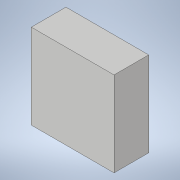
# Autodesk Inventor part: Battery
Saved by Autodesk Inventor 2021 (Build 250183000, 183)
## iProperties
Created: 2020-10-20
Part Number: Battery
Material: Generic
Document SubType Name: Modeling
Designer: Jawal
Density: 1 g/cm^3
Appearance: Default
Author: Jawal
Autodesk Inventor part; units mm, degrees
ref_plane "YZ Plane" through (0, 0, 0) normal (1, 0, 0) x (0, 1, 0)
ref_plane "XZ Plane" through (0, 0, 0) normal (0, 1, 0) x (-1, 0, 0)
ref_plane "XY Plane" through (0, 0, 0) normal (0, 0, 1) x (1, 0, 0)
sketch "Sketch2" plane through (0, 0, 0) normal (0, 0, 1) x (1, 0, 0)
  line L0 (0, 0) -> (135, 0)
  line L1 (135, 0) -> (135, 139)
  line L2 (135, 139) -> (0, 139)
  line L3 (0, 139) -> (0, 0)
  dimension "d4" = 135
  dimension "d5" = 139
  constraints: 8 end point, 2 parallel, 1 horizontal, 1 perpendicular
  measures "d4" distance of L2.end L1.end
  measures "d5" distance of L2.end L0.start
extrude "Extrusion2" add sketch "Sketch2" along normal blind 75
sketch "Sketch3" plane through (135, 0, 0) normal (1, 0, 0) x (0, 0, -1)
  line L0 (0, 139) -> (-75, 139) projected
  line L1 (-75, 139) -> (0, 139)
  line L2 (0, 139) -> (0, 0)
  line L3 (0, 0) -> (-75, 0)
  line L4 (-75, 0) -> (-75, 139)
  constraints: 8 end point, 2 parallel, 1 horizontal, 1 perpendicular
extrude "Extrusion3" add sketch "Sketch3" along normal blind 20
sketch "Sketch4" plane through (0, 139, 75) normal (0, 1, 0) x (1, 0, 0)
  line L0 (0, 0) -> (155, 0) projected
  line L1 (0, 75) -> (155, 75)
  line L2 (155, 75) -> (155, 0)
  line L3 (155, 0) -> (0, 0)
  line L4 (0, 0) -> (0, 75)
  constraints: 8 end point, 2 parallel, 1 horizontal, 1 perpendicular
extrude "Extrusion4" add sketch "Sketch4" along normal blind 20
sketch "Sketch5" plane through (0, 0, 0) normal (0, 0, -1) x (-1, 0, 0)
  line L0 (-155, 0) -> (-155, 159) projected
  line L1 (-155, 159) -> (0, 159)
  line L2 (0, 159) -> (0, 0)
  line L3 (0, 0) -> (-155, 0)
  line L4 (-155, 0) -> (-155, 159)
  constraints: 8 end point, 2 parallel, 1 horizontal, 1 perpendicular
extrude "Extrusion5" cut sketch "Sketch5" against normal blind 10
body "Solid2"
